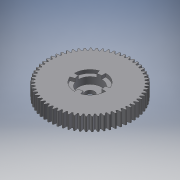
# Autodesk Inventor part: gear 1 clutch
Saved by Autodesk Inventor 2017 (Build 210142000, 142)
## iProperties
Created: 2018-04-17
Part Number: gear 1 clutch
Material: Generic
Document SubType Name: Modeling
Designer: RKL
Density: 1 g/cm^3
Appearance: Default
Author: RKL
Autodesk Inventor part; units mm, degrees
ref_plane "YZ Plane" through (0, 0, 0) normal (1, 0, 0) x (0, 1, 0)
ref_plane "XZ Plane" through (0, 0, 0) normal (0, 1, 0) x (-1, 0, 0)
ref_plane "XY Plane" through (0, 0, 0) normal (0, 0, 1) x (1, 0, 0)
sketch "Sketch1" plane through (0, 0, 0) normal (0, 0, 1) x (1, 0, 0)
  spline S0 degree 3 poles (-2.567, 62.9477) (-2.3592, 62.5224) (-1.9438, 61.6718) (-1.5124, 60.5697) (-1.2035, 59.6741) (-1.058, 59.1022) (-0.9261, 58.707) (-0.7985, 58.5062) (-0.6731, 58.3788) (-0.5232, 58.282) (-0.2987, 58.1981) (0, 58.2139) (0.2987, 58.1981) (0.5232, 58.282) (0.6731, 58.3788) (0.7985, 58.5062) (0.9261, 58.707) (1.058, 59.1022) (1.2035, 59.6741) (1.5124, 60.5697) (1.9438, 61.6718) (2.3592, 62.5224) (2.567, 62.9477) knots 0 0 0 0 0.141934 0.283863 0.354836 0.425808 0.461213 0.478956 0.496701 0.514413 0.532148 0.567547 0.602946 0.620681 0.638392 0.656138 0.673881 0.709286 0.780258 0.851231 0.99316 1.135094 1.135094 1.135094 1.135094
  circle A0 centre (0, 0) radius 58.2076 construction
  circle A1 centre (0, 0) radius 57.3212 construction
  circle A2 centre (0, 0) radius 61 construction
  circle A3 centre (0, 0) radius 63
  point P0 (-1.9614, 61.664)
  point P1 (-1.4382, 60.3447)
  point P2 (-1.213, 59.6716)
  point P3 (-1.0173, 58.9894)
  point P4 (-0.8899, 58.6591)
  point P5 (-0.7935, 58.5101)
  point P6 (-0.6689, 58.3838)
  point P7 (-0.5201, 58.2877)
  point P8 (-0.3535, 58.2271)
  point P9 (0, 58.2076)
  point P10 (0.3535, 58.2271)
  point P11 (0.5201, 58.2877)
  point P12 (0.6689, 58.3838)
  point P13 (0.7935, 58.5101)
  point P14 (0.8899, 58.6591)
  point P15 (1.0173, 58.9894)
  point P16 (1.213, 59.6716)
  point P17 (1.4382, 60.3447)
  point P18 (1.9614, 61.664)
  constraints: 4 centre point, 2 point on circle, 47 other
extrude "Extrusion1" add sketch "Sketch1" against normal blind 20
extrude "Extrusion2" cut sketch "Sketch1" against normal through all contours A3 S0 picked at (-0.1281, 61.0906)
pattern_circular "Circular Pattern1" count 61 over 360 about axis through (0, 0, 0) along (0, 0, -1) of "Extrusion2"
sketch "Sketch2" plane through (0, 0, 0) normal (0, 0, 1) x (1, 0, 0)
  circle A0 centre (0, 0) radius 6.75
  dimension "d7" = 13.5
  constraints: 1 centre point, 1 coincident
  measures "d7" diameter of A0
extrude "Extrusion3" cut sketch "Sketch2" against normal through all
sketch "Sketch3" plane through (0, 0, 0) normal (0, 0, 1) x (1, 0, 0)
  circle A0 centre (0, 0) radius 17.5
  dimension "d10" = 35
  constraints: 1 centre point, 1 coincident
  measures "d10" diameter of A0
extrude "Extrusion4" cut sketch "Sketch3" against normal blind 15
sketch "Sketch4" plane through (0, 0, 0) normal (0, 0, 1) x (1, 0, 0)
  circle A0 centre (0, 0) radius 17.5 construction
  line L0 (0, 0) -> (0, 17.5) construction
  line L1 (0, 17.5) -> (0, 23.5)
  arc A1 (22.0828, 8.0375) -> (0, 23.5) centre (0, 0) ccw
  arc A2 (16.4446, 5.9854) -> (0, 17.5) centre (0, 0) ccw
  line L2 (22.0828, 8.0375) -> (16.4446, 5.9854)
  dimension "d13" = 6
  dimension "d14" = 70
  constraints: 6 end point, 4 point on circle, 2 centre point, 2 coincident, 1 line through centre, 1 point on line, 1 vertical, 1 vertical alignment, 1 other
  measures "d13" distance of L0.end L1.end
  measures "d14" angle of L2 L1
extrude "Extrusion5" cut sketch "Sketch4" against normal blind 5
pattern_circular "Circular Pattern2" count 4 over 360 about axis through (0, 0, 0) along (0, 0, -1) of "Extrusion5"
equation "\"d0\" = FaceWidth"
equation "\"Module\" = 2"
equation "\"PressureAngle\" = 20deg"
equation "\"UnitProfileClearance\" = 0.25"
equation "\"UnitRoundRadius\" = 0.3335"
equation "\"HeadDiameter\" = 126"
equation "\"RootDiameter\" = 116.41524"
equation "\"BaseDiameter\" = 114.6425"
equation "\"PitchDiameter\" = 122"
equation "\"FaceWidth\" = 20"
equation "\"HelixAngle\" = 0"
equation "\"UnitCorrection\" = 0"
equation "\"UnitAddendumModification\" = 0"
equation "\"CircularPitch\" = 6.283185"
equation "\"UnitBacklashShift\" = -0.14619"
equation "\"TotalToolShift\" = -0.29238"
equation "\"IsInternal\" = 0"
body "Solid1"
